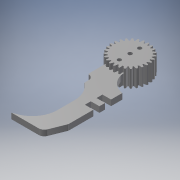
# Autodesk Inventor part: Spur Gear2
Saved by Autodesk Inventor 2017 (Build 210142000, 142)
## iProperties
Created: 2017-05-25
Part Number: Spur Gear2
Material: Steel
Document SubType Name: Modeling
Designer: Andres Celi
Categories: <?xml version="1.0" encoding="UTF-16"?> <MemberInstance><Categories><FamilyTemplate><FamilyTemplateParameter ValueType="xs:double" Id="1" ObjectReferenceKey="da_z" ObjectType="kUserParameterObject"/><FamilyTemplateParameter ValueType="xs:double" Id="2" ObjectReferenceKey="da_b" ObjectType="kUserParameterObject"/><FamilyTemplateParameter ValueType="xs:double" Id="3" ObjectReferenceKey="da_beta" ObjectType="kUserParameterObject"/><FamilyTemplateParameter ValueType="xs:double" Id="4" ObjectReferenceKey="da_da" ObjectType="kUserParameterObject"/><FamilyTemplateParameter ValueType="xs:double" Id="5" ObjectReferenceKey="da_aw" ObjectType="kUserParameterObject"/><FamilyTemplateParameter ValueType="xs:string" Id="6" ObjectReferenceKey="EAIAABAAAACIAQAAAAAAAIAAAAAAAAAA" ObjectType="83910656" SubObjectId="SurfaceGeometry"/></FamilyTemplate><ParamToTemplateMap><ParamToTemplate CategoryParameter="//CategoryParameter[@InternalName='046C89C9-8512-4d59-83FE-43B91F4F132A']" TemplateParameter="1"/><ParamToTemplate CategoryParameter="//CategoryParameter[@InternalName='2552DF32-E462-4b46-AEBF-C6C7768E72AC']" TemplateParameter="2"/><ParamToTemplate CategoryParameter="//CategoryParameter[@InternalName='C9EE641D-15FC-4fae-A226-E94C4372FDD7']" TemplateParameter="3"/><ParamToTemplate><ParamToTemplate CategoryParameter="//CategoryParameter[@InternalName='00B6519A-459B-49c7-AD84-2E56D39A5744']" ConstantValue="0.086878"/></ParamToTemplate><ParamToTemplate><ParamToTemplate CategoryParameter="//CategoryParameter[@InternalName='04B31F0E-C7A6-4894-AA32-9629BEFACF47']" ConstantValue="1.000000"/></ParamToTemplate><ParamToTemplate><ParamToTemplate CategoryParameter="//CategoryParameter[@InternalName='43CBEC2E-7847-49e7-A936-2F7889FCB2D9']" ConstantValue="0.250000"/></ParamToTemplate><ParamToTemplate><ParamToTemplate CategoryParameter="//CategoryParameter[@InternalName='B1EFC894-105D-4ebd-86BF-FA20ED196853']" ConstantValue="0.350000"/></ParamToTemplate><ParamToTemplate><ParamToTemplate CategoryParameter="//CategoryParameter[@InternalName='51175063-3D10-4879-93E8-6246FE8B403D']" ConstantValue="2060000000.000000"/></ParamToTemplate><ParamToTemplate><ParamToTemplate CategoryParameter="//CategoryParameter[@InternalName='A3A52E27-4454-46a9-B0BD-C932399B70AF']" ConstantValue="0.300000"/></ParamToTemplate><ParamToTemplate><ParamToTemplate CategoryParameter="//CategoryParameter[@InternalName='91B76062-C214-41d9-B1B9-14D2AB99603D']" ConstantValue="0.112500"/></ParamToTemplate><ParamToTemplate><ParamToTemplate CategoryParameter="//CategoryParameter[@InternalName='374E806E-8B8A-4dda-A9AA-1039D6500AD2']" ConstantValue="8.888889"/></ParamToTemplate><ParamToTemplate><ParamToTemplate CategoryParameter="//CategoryParameter[@InternalName='2D373A89-B862-43d6-8D0B-0CBF12AB9F6C']" ConstantValue="0.349066"/></ParamToTemplate><ParamToTemplate CategoryParameter="//CategoryParameter[@InternalName='37777632-D6A2-4fac-9D53-DB8ACD95C989']" TemplateParameter="4"/><ParamToTemplate CategoryParameter="//CategoryParameter[@InternalName='FD1017F1-B727-4f7e-9707-0F86F1FF9423']" TemplateParameter="5"/><ParamToTemplate><ParamToTemplate CategoryParameter="//CategoryParameter[@InternalName='9E1B4470-B2D3-4ff1-B813-535BB4CDF51A']" ConstantValue="3520000.000000"/></ParamToTemplate><ParamToTemplate><ParamToTemplate CategoryParameter="//CategoryParameter[@InternalName='F8452263-BFF6-458c-9FB1-07C4B99E95CD']" ConstantValue="11400000.000000"/></ParamToTemplate><ParamToTemplate><ParamToTemplate CategoryParameter="//CategoryParameter[@InternalName='3E3BB259-FD49-497f-8171-6EBC954A3479']" ConstantValue="2.000000"/></ParamToTemplate><ParamToTemplate CategoryParameter="//CategoryParameter[@InternalName='27C3BAF2-7550-4e4b-AE2C-0DB134B7D9B7']" TemplateParameter="6"/></ParamToTemplateMap><Category DisplayName="Gear" InternalName="DC85795E-93AB-48d5-8EEE-5A27447B64BD" Mnemonic="Gear"><CategoryParameter DisplayName="z" InternalName="046C89C9-8512-4d59-83FE-43B91F4F132A" Mnemonic="z"/><CategoryParameter DisplayName="b" InternalName="2552DF32-E462-4b46-AEBF-C6C7768E72AC" Mnemonic="b"/><CategoryParameter DisplayName="||b|" InternalName="C9EE641D-15FC-4fae-A226-E94C4372FDD7" Mnemonic="beta"/><CategoryParameter DisplayName="x" InternalName="00B6519A-459B-49c7-AD84-2E56D39A5744" Mnemonic="x"/><CategoryParameter DisplayName="a*" InternalName="04B31F0E-C7A6-4894-AA32-9629BEFACF47" Mnemonic="a"/><CategoryParameter DisplayName="c*" InternalName="43CBEC2E-7847-49e7-A936-2F7889FCB2D9" Mnemonic="c"/><CategoryParameter DisplayName="r|.f|*" InternalName="B1EFC894-105D-4ebd-86BF-FA20ED196853" Mnemonic="rf"/><CategoryParameter DisplayName="E" InternalName="51175063-3D10-4879-93E8-6246FE8B403D" Mnemonic="E"/><CategoryParameter DisplayName="||m|" InternalName="A3A52E27-4454-46a9-B0BD-C932399B70AF" Mnemonic="mi"/><Category DisplayName="SpurGear" InternalName="26C5A22E-A91E-4dfd-A3B3-23CCAFAE1764" Mnemonic="SpurGear"><CategoryParameter DisplayName="m" InternalName="91B76062-C214-41d9-B1B9-14D2AB99603D" Mnemonic="m"/><CategoryParameter DisplayName="P" InternalName="374E806E-8B8A-4dda-A9AA-1039D6500AD2" Mnemonic="PP"/><CategoryParameter DisplayName="||a|" InternalName="2D373A89-B862-43d6-8D0B-0CBF12AB9F6C" Mnemonic="alpha"/><CategoryParameter DisplayName="d|.a|" InternalName="37777632-D6A2-4fac-9D53-DB8ACD95C989" Mnemonic="da"/><CategoryParameter DisplayName="a|.w|" InternalName="FD1017F1-B727-4f7e-9707-0F86F1FF9423" Mnemonic="aw"/><CategoryParameter DisplayName="||s||.Flim|" InternalName="9E1B4470-B2D3-4ff1-B813-535BB4CDF51A" Mnemonic="sFlim"/><CategoryParameter DisplayName="||s||.Hlim|" InternalName="F8452263-BFF6-458c-9FB1-07C4B99E95CD" Mnemonic="sHlim"/><CategoryParameter DisplayName="type" InternalName="3E3BB259-FD49-497f-8171-6EBC954A3479" Mnemonic="type"/><CategoryParameter DisplayName="PitchDiameter" InternalName="27C3BAF2-7550-4e4b-AE2C-0DB134B7D9B7" Mnemonic="IDS_PITCHDIAM"/></Category></Category></Categories></MemberInstance>
Density: 1 g/cm^3
Appearance: Steel
CustomPartVersion: 1
Author: Andres Celi
Autodesk Inventor part; units mm, degrees
ref_plane "YZ Plane" through (0, 0, 0) normal (1, 0, 0) x (0, 1, 0)
ref_plane "XZ Plane" through (0, 0, 0) normal (0, 1, 0) x (-1, 0, 0)
ref_plane "XY Plane" through (0, 0, 0) normal (0, 0, 1) x (1, 0, 0)
sketch "Sketch1" plane through (0, 0, 0) normal (0, 0, 1) x (1, 0, 0)
  circle A0 centre (0, 0) radius 16.4059
  dimension "d0" = 32.8118
  constraints: 1 centre point
  measures "d0" diameter of A0
extrude "Extrusion1" add sketch "Sketch1" along normal blind 15
ref_plane "Work Plane2" through (0, 0, 7.5) normal (0, 0, 1) x (1, 0, 0)
sketch "Sketch2" plane through (0, 0, 0) normal (0, 0, -1) x (-1, 0, 0)
  circle A0 centre (0, 0) radius 16.4059 projected
  circle A1 centre (0, 0) radius 15.283
  dimension "d3" = 30.566
  constraints: 1 centre point, 1 coincident
  measures "d3" diameter of A1
surface extrude "Pitch Diameter" sketch "Sketch2" against normal through all shown no curves A1
ref_plane "Work Plane8" through (0, 0, 0) normal (0.9932384, 0.1160929, 0) x (0, 0, 1)
ref_plane "Work Plane9" through (0, 0, 0) normal (1, 0, 0) x (0, 1, 0)
spur gear teeth "Spur Gear" teeth 27 pitch diameter 30.375 tip diameter 32.8118 root diameter 27.758 face width 15 start plane through (0, 0, 0) normal (0, 0, -1) x (-1, 0, 0)
sketch "Sketch3" plane through (0, 0, 15) normal (0, 0, 1) x (1, 0, 0)
  circle A0 centre (0, 0) radius 1.75
  dimension "d49" = 3.5
  constraints: 1 centre point, 1 coincident
  measures "d49" diameter of A0
extrude "Extrusion2" cut sketch "Sketch3" against normal blind 21
sketch "Sketch4" plane through (0, 0, 15) normal (0, 0, 1) x (1, 0, 0)
  circle A0 centre (0, 8.3245) radius 1.65
  circle A1 centre (0, -9.4344) radius 1.65
  point P0 (0, 0)
  dimension "d52" = 3.3
  dimension "d53" = 3.3
  constraints: 2 centre point
  measures "d52" diameter of A0
  measures "d53" diameter of A1
extrude "Extrusion3" cut sketch "Sketch4" against normal blind 20
ref_plane "Work Plane11" through (0, 0, 10) normal (0, 0, 1) x (1, 0, 0)
sketch "Sketch5" plane through (0, 0, 10) normal (0, 0, 1) x (1, 0, 0)
  line L0 (21.5, -53.588) -> (21.5, -74.6259)
  arc A0 (21.1457, -76.4745) -> (21.5, -74.6259) centre (16.5, -74.6259) ccw
  line L1 (6, -69.75) -> (6, -54.75)
  line L2 (16.3216, -88.5985) -> (21.1457, -76.4745)
  arc A1 (11.6759, -91.75) -> (16.3216, -88.5985) centre (11.6759, -86.75) ccw
  arc A2 (-9.9013, -90.8878) -> (6, -69.75) centre (-16, -69.75) ccw
  line L3 (-12.207, -91.75) -> (11.6759, -91.75)
  line L4 (-9.9013, -90.8878) -> (-12.207, -91.75)
  line L5 (14, -53.588) -> (21.5, -53.588)
  line L6 (14, -48.388) -> (14, -53.588)
  line L7 (21.5, -48.388) -> (14, -48.388)
  arc A3 (6, -54.75) -> (-3, -37.0018) centre (-16, -54.75) ccw
  line L8 (14, -43.388) -> (21.5, -43.388)
  line L9 (21.5, -43.388) -> (21.5, -48.388)
  line L10 (-3, -37.0018) -> (-3, -33.0018)
  line L11 (14, -38.188) -> (14, -43.388)
  line L12 (21.5, -38.188) -> (14, -38.188)
  line L13 (-8, -28.0018) -> (-8, -1.75)
  line L14 (-8, -1.75) -> (7, -1.75)
  line L15 (7, -1.75) -> (7, -11.4872)
  line L16 (21.5, -28.4872) -> (21.5, -38.188)
  arc A4 (7, -11.4872) -> (21.5, -28.3024) centre (24, -11.4872) ccw
  arc A5 (-3, -33.0018) -> (-7, -29.0018) centre (-7, -33.0018) ccw
  arc A6 (-8, -28.0018) -> (-7, -29.0018) centre (-7, -28.0018) ccw
  line L17 (21.5, -28.4872) -> (21.5, -28.3024)
  point P0 (0, 0)
  point P1 (-16, -91.75)
  point P2 (-16, -97.3941)
  point P3 (-3, -29.0018)
  dimension "d57" = 22
  dimension "d58" = 90
  dimension "d59" = 0
  dimension "d60" = 15
  dimension "d61" = 0
  dimension "d62" = 13
  dimension "d63" = 22
  dimension "d64" = 8
  dimension "d65" = 37
  dimension "d66" = 5
  dimension "d67" = 12.1241
  dimension "d68" = 5.2
  dimension "d69" = 5.2
  dimension "d70" = 5
  dimension "d71" = 17
  dimension "d72" = 4
  dimension "d73" = 90
  dimension "d74" = 8
  dimension "d75" = 15
  dimension "d76" = 1
  dimension "d77" = 158.303
  dimension "d78" = 110.503
  dimension "d79" = 7.5
  dimension "d80" = 53.562
  dimension "d81" = 28.8665
  dimension "d82" = 1.3285
  dimension "d83" = 21.3742
  dimension "d84" = 17.412
  dimension "d85" = 1.75
  dimension "d86" = 26.2518
  dimension "d87" = 8
  constraints: 36 end point, 14 point on circle, 11 tangent, 7 centre point, 7 perpendicular, 7 vertical, 4 point on line, 2 horizontal, 1 equal radius, 1 parallel, 6 other
  measures "d57" radius of A2
  measures "d59" horizontal distance of point (-16, -97.394) A2.centre
  measures "d60" distance of L1.start L1.end
  measures "d61" horizontal distance of point (-16, -97.394) A3.centre
  measures "d62" horizontal distance of A3.centre L10.start
  measures "d63" radius of A3
  measures "d64" distance of L10.start point (-3, -29.002)
  measures "d65" distance from line of L2 A2.centre
  measures "d66" radius of A0
  measures "d67" vertical distance of L2.start L2.end
  measures "d68" distance between parallel lines of L8 L12
  measures "d69" distance between parallel lines of L5 L7
  measures "d70" distance between parallel lines of L8 L7
  measures "d71" radius of A4
  measures "d72" radius of A5
  measures "d73" distance between parallel lines of L3 L14
  measures "d74" distance from line of L13 point (-16, -91.75)
  measures "d75" distance of L13.end L14.end
  measures "d76" radius of A6
  measures "d77" angle of L0 L2
  measures "d78" angle of L4 L0
  measures "d79" distance between parallel lines of L11 L0
  measures "d80" distance between parallel lines of L12 L3
  measures "d81" distance from line of point (-16, -91.75) L2
  measures "d82" distance from line of point (-16, -91.75) L4
  measures "d83" distance from line of A4.centre L2
  measures "d84" distance from line of L16.start L2
  measures "d85" distance from line of L14 point (0, 0)
  measures "d86" distance of L13.start L13.end
  measures "d87" distance from line of point (0, 0) L13
extrude "Extrusion4" add sketch "Sketch5" against normal blind 5
sketch "Sketch6" plane through (0, 0, 15) normal (0, 0, 1) x (1, 0, 0)
  circle A0 centre (0, 0) radius 1.75
  dimension "d90" = 3.5
  constraints: 1 centre point, 1 coincident
  measures "d90" diameter of A0
extrude "Extrusion5" cut sketch "Sketch6" against normal blind 20
sketch "Sketch7" plane through (0, 0, 15) normal (0, 0, 1) x (1, 0, 0)
  circle A0 centre (0, -9.4344) radius 1.65 projected
  circle A1 centre (0, -9.4344) radius 1.65
  point P0 (0, 0)
  constraints: 1 centre point, 1 coincident
extrude "Extrusion6" cut sketch "Sketch7" against normal blind 20
equation "\"d0\" = da_da"
equation "\"d1\" = da_b"
equation "\"d3\" = da_dw"
equation "\"da_da\" = 32.811764"
equation "\"da_b\" = 15"
equation "\"da_dw\" = 30.566038"
body "Solid1"
body "Srf1"
